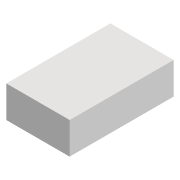
# Autodesk Inventor part: Part79
Saved by Autodesk Inventor 2020.5 (Build 245400000, 400)
## iProperties
Created: 2022-11-26
Part Number: Part79
Material: 一般
Document SubType Name: Modeling
Designer: Administrator
Density: 1 g/cm^3
Appearance: 既定
Author: Administrator
Autodesk Inventor part; units mm, degrees
ref_plane "YZ Plane" through (0, 0, 0) normal (1, 0, 0) x (0, 1, 0)
ref_plane "XZ Plane" through (0, 0, 0) normal (0, 1, 0) x (-1, 0, 0)
ref_plane "XY Plane" through (0, 0, 0) normal (0, 0, 1) x (1, 0, 0)
sketch "スケッチ1" plane through (0, 0, 0) normal (0, 0, 1) x (1, 0, 0)
  line L0 (120.9986, 72.869) -> (120.9986, -75.131) projected
  line L1 (-39.0005, 72.869) -> (9.2493, 72.869) projected
  line L2 (-39.0005, -75.131) -> (-39.0005, 72.869) projected
  line L3 (9.2493, 72.869) -> (9.2493, 60.119) projected
  arc A0 (9.2493, 60.119) -> (39.2493, 60.119) centre (24.2493, 60.119) ccw projected
  line L4 (39.2493, 60.119) -> (39.2493, 72.869) projected
  line L5 (39.2493, 72.869) -> (120.9986, 72.869) projected
  line L6 (120.9986, -75.131) -> (-39.0005, -75.131) projected
  line L7 (105.9986, -75.131) -> (-24.0005, -75.131)
  line L8 (-24.0005, -75.131) -> (-24.0005, -15.131)
  line L9 (-24.0005, -15.131) -> (105.9986, -15.131)
  line L10 (105.9986, -15.131) -> (105.9986, -75.131)
  point P0 (0, 0)
  point P1 (-24.0005, -75.131)
  point P2 (105.9986, -75.131)
  dimension "d8" = 15
  dimension "d9" = 15
  dimension "d10" = 60
  dimension "d11" = 0
  constraints: 8 end point, 2 parallel, 1 horizontal, 1 perpendicular
  measures "d8" distance between parallel lines of L0 L10
  measures "d9" distance between parallel lines of L2 L8
  measures "d10" distance between parallel lines of L9 L7
  measures "d11" distance between parallel lines of L7 L6
extrude "押し出し1" add sketch "スケッチ1" along normal blind 197 contours L6 L8 L9 L10
